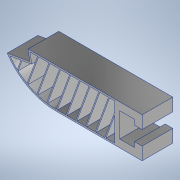
# Autodesk Inventor part: Finray_9_Kerbe_10deg_20deg10inf_PLA
Saved by Autodesk Inventor 2022 (Build 260153000, 153)
## iProperties
Created: 2022-02-28
Part Number: Finray_9_Kerbe_10deg_20deg10inf_PLA
Material: Generic
Document SubType Name: Modeling
Designer: richa
Density: 1 g/cm^3
Appearance: Aluminum - Flat
Author: richa
Autodesk Inventor part; units mm, degrees
ref_plane "YZ Plane" through (0, 0, 0) normal (1, 0, 0) x (0, 1, 0)
ref_plane "XZ Plane" through (0, 0, 0) normal (0, 1, 0) x (-1, 0, 0)
ref_plane "XY Plane" through (0, 0, 0) normal (0, 0, 1) x (1, 0, 0)
sketch "Sketch5" plane through (0, 0, 0) normal (0, 0, 1) x (1, 0, 0)
  line L0 (52.8, -15.6) -> (52.8, -10.6)
  line L1 (52.8, -10.6) -> (49.8, -10.6)
  line L2 (49.8, -10.6) -> (49.8, -12.6)
  line L3 (44, -12.6) -> (44, -3)
  line L4 (49.8, -3) -> (49.8, -5)
  line L5 (49.8, -5) -> (52.8, -5)
  line L6 (52.8, -5) -> (52.8, 0)
  line L7 (52.8, 0) -> (7.8, 0)
  line L8 (44, -3) -> (49.8, -3)
  line L9 (44, -12.6) -> (49.8, -12.6)
  line L10 (52.8, -15.6) -> (7.8, -15.6)
  line L11 (7.8, -15.6) -> (0, -15.6)
  line L12 (0, -15.6) -> (0, 0)
  line L13 (0, 0) -> (7.8, 0)
  point P0 (7.8, 0)
  dimension "d41" = 5.8
  dimension "d48" = 44
  dimension "d50" = 3
  dimension "d63" = 45
  dimension "d71" = 0
  dimension "d87" = 5.6
  dimension "d88" = 9.6
  dimension "d97" = 15.6
  constraints: 28 end point, 8 perpendicular, 4 collinear, 3 parallel, 2 horizontal, 1 vertical
  measures "d41" distance between parallel lines of L2 L3
  measures "d48" distance from line of L3 L12.end
  measures "d50" distance of L4.end L5.end
  measures "d63" distance of L0.start L10.end
  measures "d71" distance from line of L12.end L7
  measures "d87" distance from line of L0.end L5
  measures "d88" distance of L3.start L3.end
  measures "d97" distance of L11.end L12.end
extrude "Extrusion2" add sketch "Sketch5" along normal blind 12
sketch "Sketch8" plane through (0, 0, 0) normal (0, 0, -1) x (-1, 0, 0)
  line L0 (-8.1687, 0) -> (-8.8633, -3.9392)
  line L1 (-7.8, 0) -> (-1.143, 0) construction
  line L2 (0, -5.5021) -> (-8.8633, -3.9392)
  line L3 (-7.8, 0) -> (-8.1687, 0)
  line L4 (0, 0) -> (0, -15.6) projected
  line L5 (-52.8, 0) -> (0, 0) projected
  line L6 (-7.8, 0) -> (0, 0)
  line L7 (0, 0) -> (0, -5.5021)
  dimension "d80" = 100
  dimension "d95" = 4
  dimension "d96" = 9
  constraints: 12 end point, 2 collinear, 2 perpendicular, 1 horizontal, 1 point on line
  measures "d80" angle of L0 L1
  measures "d95" distance of L0.start L0.end
  measures "d96" distance of L2.start L0.end
extrude "Extrusion5" cut sketch "Sketch8" against normal through all
fillet "Fillet2" radius 23 1 edges at (0, -15.6, 6)
shell "Shell1" thickness 0.62 removed faces 1 at (23.9679, -7.5131, 12)
sketch "Sketch13" plane through (0, 0, 12) normal (0, 0, 1) x (1, 0, 0)
  line L0 (19.0404, -15.6) -> (52.8, -15.6) projected
  line L1 (42.0526, -15.6) -> (42.0526, 0)
  line L2 (52.8, 0) -> (8.1687, 0) projected
  line L3 (52.8, 0) -> (8.1687, 0) projected
  line L4 (52.8, -5) -> (52.8, 0) projected
  line L5 (49.8, -5) -> (52.8, -5) projected
  line L6 (49.8, -3) -> (49.8, -5) projected
  line L7 (44, -3) -> (49.8, -3) projected
  line L8 (44, -12.6) -> (44, -3) projected
  line L9 (49.8, -12.6) -> (44, -12.6) projected
  line L10 (49.8, -10.6) -> (49.8, -12.6) projected
  line L11 (52.8, -10.6) -> (49.8, -10.6) projected
  line L12 (52.8, -15.6) -> (52.8, -10.6) projected
  line L13 (42.0526, 0) -> (52.8, 0)
  line L14 (52.8, -5) -> (52.8, 0) projected
  line L15 (52.8, -5) -> (52.8, 0)
  line L16 (52.8, 0) -> (52.8, -5)
  line L17 (44, -12.6) -> (44, -3) projected
  line L18 (44, -3) -> (44, -12.6)
  line L19 (49.8, -12.6) -> (44, -12.6) projected
  line L20 (44, -12.6) -> (49.8, -12.6)
  line L21 (43.38, -13.22) -> (50.42, -13.22) projected
  line L22 (52.8, -10.6) -> (52.8, -15.6)
  line L23 (52.8, -15.6) -> (42.0526, -15.6)
  line L24 (44, -3) -> (49.8, -3) projected
  line L25 (44, -3) -> (49.8, -3)
  line L26 (49.8, -3) -> (49.8, -5)
  line L27 (49.8, -5) -> (52.8, -5)
  line L28 (52.8, -10.6) -> (49.8, -10.6)
  line L29 (49.8, -10.6) -> (49.8, -12.6)
  point P0 (0, 0)
  dimension "d102" = 10.7474
  constraints: 26 end point, 10 collinear, 2 point on line, 2 vertical, 1 parallel
  measures "d102" distance between parallel lines of L4 L1
extrude "Extrusion7" add sketch "Sketch13" against normal blind 12
sketch "Sketch14" plane through (8.9076, -0.62, 0.62) normal (0, 0, 1) x (1, 0, 0)
  line L0 (33.145, -14.36) -> (33.145, 0) projected
  line L1 (33.145, 0) -> (0, 0) projected
  line L2 (0.6739, -3.8221) -> (0, 0) projected
  line L3 (-7.835, -5.3225) -> (0.6739, -3.8221) projected
  arc A0 (-7.835, -5.3225) -> (10.1328, -14.36) centre (10.1328, 8.02) ccw projected
  line L4 (10.1328, -14.36) -> (33.145, -14.36) projected
  point P0 (-8.9076, 0.62)
extrude "Extrusion8" cut sketch "Sketch14" against normal blind 12
sketch "Sketch15" plane through (0, 0, 12) normal (0, 0, 1) x (1, 0, 0)
  line L0 (42.0526, -0.62) -> (8.9076, -0.62) construction
  line L1 (19.0404, -14.98) -> (42.0526, -14.98) projected
  line L2 (43.5165, -0.49) -> (43.8736, -0.62)
  line L3 (43.8736, -0.62) -> (38.5997, -15.11)
  line L4 (38.5997, -15.11) -> (38.2426, -14.98)
  line L5 (38.2426, -14.98) -> (43.5165, -0.49)
  arc A0 (1.0726, -5.9425) -> (19.0404, -14.98) centre (19.0404, 7.4) ccw projected
  line L6 (42.0526, -0.62) -> (42.0526, -14.98) projected
  line L7 (1.0726, -5.9425) -> (9.5815, -4.4421) projected
  arc A1 (0, -5.5021) -> (19.0404, -15.6) centre (19.0404, 7.4) ccw projected
  line L8 (42.0526, -14.98) -> (19.0404, -14.98) projected
  line L9 (8.9076, -0.62) -> (42.0526, -0.62) projected
  line L10 (40.0636, -0.62) -> (34.837, -14.98)
  line L11 (39.6592, -0.62) -> (34.4326, -14.98)
  line L12 (32.4436, -0.62) -> (27.217, -14.98)
  line L13 (32.0392, -0.62) -> (26.8126, -14.98)
  line L14 (28.6336, -0.62) -> (23.407, -14.98)
  line L15 (28.2292, -0.62) -> (23.0026, -14.98)
  line L16 (24.8236, -0.62) -> (19.597, -14.98)
  line L17 (24.4192, -0.62) -> (19.1926, -14.98)
  line L18 (20.9041, -0.62) -> (15.7652, -14.739)
  line L19 (16.7367, -0.62) -> (11.9319, -13.8211)
  line L20 (16.3323, -0.62) -> (11.5726, -13.6973)
  line L21 (12.2837, -0.62) -> (8.0973, -12.1221)
  line L22 (11.8794, -0.62) -> (7.7626, -11.9307)
  line L23 (5.8217, -5.1051) -> (4.2575, -9.4027)
  line L24 (5.3896, -5.1813) -> (3.9526, -9.1295)
  line L25 (20.4997, -0.62) -> (15.3826, -14.6791)
  line L26 (36.2536, -0.62) -> (31.027, -14.98)
  line L27 (35.8492, -0.62) -> (30.6226, -14.98)
  point P0 (0, 0)
  point P1 (38.2426, -14.98)
  point P2 (38.647, -14.98)
  point P3 (27.217, -14.98)
  point P4 (23.407, -14.98)
  point P5 (19.597, -14.98)
  dimension "d105" = 0.38
  dimension "d129" = 3.81
  dimension "d130" = 110
  dimension "d132" = 110
  dimension "d133" = 0.38
  dimension "d135" = 0.38
  dimension "d136" = 0.38
  dimension "d137" = 0.38
  dimension "d138" = 0.38
  dimension "d139" = 0.38
  dimension "d140" = 0.38
  dimension "d141" = 0.38
  dimension "d142" = 3.81
  dimension "d143" = 0.38
  dimension "d144" = 3.81
  dimension "d145" = 3.81
  dimension "d146" = 3.81
  dimension "d147" = 3.81
  dimension "d148" = 3.81
  dimension "d149" = 3.81
  dimension "d150" = 3.81
  dimension "d151" = 3.81
  dimension "d152" = 110
  constraints: 44 end point, 18 parallel, 2 point on line, 1 perpendicular, 39 other
  measures "d105" distance between parallel lines of L3 L5
  measures "d129" distance from line of L6 L4.end
  measures "d130" angle of L0 L3
  measures "d132" angle of L0 L10
  measures "d133" distance between parallel lines of L10 L11
  measures "d135" distance between parallel lines of L13 L12
  measures "d136" distance between parallel lines of L15 L14
  measures "d137" distance between parallel lines of L17 L16
  measures "d138" distance between parallel lines of L25 L18
  measures "d139" distance between parallel lines of L20 L19
  measures "d140" distance between parallel lines of L22 L21
  measures "d141" distance between parallel lines of L24 L23
  measures "d142" distance of L4.end L11.end
  measures "d143" distance between parallel lines of L26 L27
  measures "d144" distance of L11.end L27.end
  measures "d145" distance of L27.end L13.end
  measures "d146" distance of L15.end L13.end
  measures "d147" distance of L15.end L17.end
  measures "d148" horizontal distance of L25.end L17.end
  measures "d149" horizontal distance of L25.end L20.end
  measures "d150" horizontal distance of L20.end L22.end
  measures "d151" horizontal distance of L22.end L24.end
  measures "d152" angle of L0 L12
extrude "Extrusion9" add sketch "Sketch15" against normal blind 12 contours L17 L9 L16 L1 | A0 L25 L9 L18 | L15 L9 L14 L1 | A0 L20 L9 L19 | L13 L9 L12 L1 | A0 L22 L9 L21 | L27 L9 L26 L1 | L11 L9 L10 L1 | L5 L6 L3 L1 | L5 L2 L3 L6 | L24 L7 L23 A0
equation "\"l1\" = 8"
equation "\"d1\" = 0.38"
body "Solid2"
